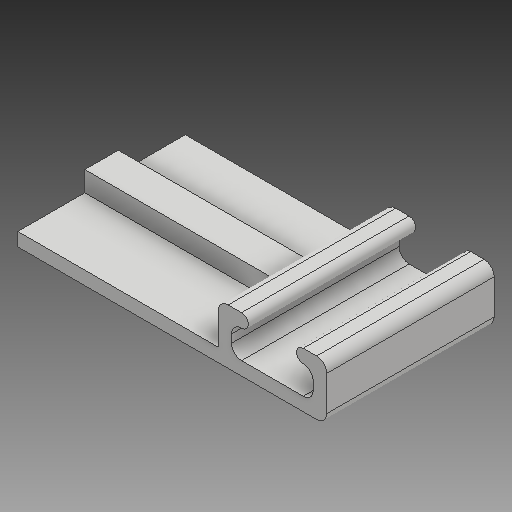
# Autodesk Inventor part: Sensor_Hook
Saved by Autodesk Inventor 2017 (Build 210142000, 142)
## iProperties
Created: 2019-10-01
Part Number: Sensor_Hook
Material: Generic
Document SubType Name: Modeling
Designer: Bear
Density: 1 g/cm^3
Appearance: Default
Author: Bear
Autodesk Inventor part; units mm, degrees
ref_plane "YZ Plane" through (0, 0, 0) normal (1, 0, 0) x (0, 1, 0)
ref_plane "XZ Plane" through (0, 0, 0) normal (0, 1, 0) x (-1, 0, 0)
ref_plane "XY Plane" through (0, 0, 0) normal (0, 0, 1) x (1, 0, 0)
sketch "Hook_Base_Skt" plane through (0, 0, 0) normal (0, 1, 0) x (-1, 0, 0)
  line L0 (4.6, -2.1) -> (-4.6, -2.1)
  line L1 (-6.1, -0.6) -> (-6.1, 0.6)
  line L2 (-4.6, 2.1) -> (4.6, 2.1) construction
  line L3 (6.1, 0.6) -> (6.1, -0.6)
  line L4 (6.1, -2.1) -> (-6.1, 2.1) construction
  line L5 (-6.1, -2.1) -> (6.1, 2.1) construction
  line L6 (8.1, -4.1) -> (-6.6, -4.1)
  line L7 (-8.1, -2.6) -> (-8.1, 2.6)
  line L8 (-6.6, 4.1) -> (-4.6, 4.1)
  line L9 (8.1, 2.6) -> (8.1, -4.1)
  line L10 (8.1, -4.1) -> (-8.1, 4.1) construction
  line L11 (-8.1, -4.1) -> (8.1, 4.1) construction
  arc A0 (6.1, 0.6) -> (4.6, 2.1) centre (4.6, 0.6) ccw
  arc A1 (4.6, -2.1) -> (6.1, -0.6) centre (4.6, -0.6) ccw
  arc A2 (-6.1, -0.6) -> (-4.6, -2.1) centre (-4.6, -0.6) ccw
  arc A3 (-4.6, 2.1) -> (-6.1, 0.6) centre (-4.6, 0.6) ccw
  arc A4 (8.1, 2.6) -> (6.6, 4.1) centre (6.6, 2.6) ccw
  arc A5 (-6.6, 4.1) -> (-8.1, 2.6) centre (-6.6, 2.6) ccw
  arc A6 (-8.1, -2.6) -> (-6.6, -4.1) centre (-6.6, -2.6) ccw
  arc A7 (4.6, 4.1) -> (4.6, 2.1) centre (4.6, 3.1) ccw
  arc A8 (-4.6, 2.1) -> (-4.6, 4.1) centre (-4.6, 3.1) ccw
  line L12 (4.6, 4.1) -> (6.6, 4.1)
  line L13 (-4.6, 4.1) -> (4.6, 4.1) construction
  point P0 (0, 0)
  dimension "d29" = 12.2
  dimension "d30" = 4.2
  dimension "d31" = 2
  dimension "d32" = 2
  dimension "d34" = 1.5
  constraints: 28 end point, 26 tangent, 18 point on circle, 14 point on line, 9 centre point, 6 equal radius, 6 parallel, 4 midpoint, 2 horizontal, 2 perpendicular
  measures "d29" distance of L4.start L5.start
  measures "d30" distance of L5.start L4.end
  measures "d31" distance between parallel lines of L9 L3
  measures "d32" distance between parallel lines of L8 L2
  measures "d34" radius of A4
extrude "Hook_Base" add sketch "Hook_Base_Skt" along normal mid plane 25
sketch "Arm_Skt" plane through (0, -12.5, 0) normal (0, -1, 0) x (1, 0, 0)
  line L0 (4.6, -2.1) -> (-4.6, -2.1) projected
  line L1 (0, -2.1) -> (-38, -2.1)
  line L2 (-38, -2.1) -> (-38, -4.1)
  line L3 (-38, -4.1) -> (0, -4.1)
  line L4 (6.6, -4.1) -> (-8.1, -4.1) projected
  line L5 (0, -4.1) -> (0, -2.1)
  point P0 (0, 0)
  dimension "d35" = 38
  constraints: 8 end point, 2 collinear, 2 perpendicular, 1 horizontal, 1 midpoint
  measures "d35" distance of L2.end L3.end
extrude "Arm" add sketch "Arm_Skt" against normal up to surface (25 mm away) from surface at 0
sketch "Arm_Rib_Skt" plane through (-38, -12.5, -2.1) normal (0, 0, 1) x (1, 0, 0)
  line L0 (38, 12.5) -> (0, 12.5) construction
  line L1 (0, 25) -> (0, 0) construction
  line L2 (29.9, 25) -> (29.9, 0) projected
  line L3 (0, 10) -> (29.9, 10)
  line L4 (29.9, 10) -> (29.9, 15)
  line L5 (29.9, 15) -> (0, 15)
  line L6 (0, 15) -> (0, 10)
  line L7 (0, 25) -> (0, 0) projected
  point P0 (0, 12.5)
  dimension "d38" = 5
  constraints: 10 end point, 3 midpoint, 2 parallel, 2 point on line, 1 horizontal, 1 perpendicular
  measures "d38" distance between parallel lines of L3 L5
extrude "Arm_Rib" add sketch "Arm_Rib_Skt" along normal blind 3
equation "\"d29\" = arm_width + 2 * clearance"
equation "\"d30\" = arm_thick + 2 * clearance"
equation "\"d31\" = hook_thick"
equation "\"d32\" = hook_thick"
equation "\"d34\" = general_fillet"
equation "\"d13\" = hook_width"
equation "\"d35\" = hole_to_border"
equation "\"d38\" = 0.2 * hook_width"
equation "\"d39\" = 1.5 * hook_thick"
equation "\"clearance\" = 0.1"
equation "\"arm_angle\" = 70deg"
equation "\"hole_diam\" = 3.1"
equation "\"hole_h_space\" = 126.2"
equation "\"hole_v_space\" = 65.65"
equation "\"arm_width\" = 12"
equation "\"arm_thick\" = 4"
equation "\"arm_rib_space\" = 1.25"
equation "\"arm_rib_thick\" = 2"
equation "\"base_width\" = 53"
equation "\"base_lenght\" = 138.2"
equation "\"general_fillet\" = 1.5"
equation "\"hole_to_border\" = 38"
equation "\"hook_width\" = 25"
equation "\"hook_thick\" = 2"
equation "\"rfid_width\" = 39.5"
equation "\"rfid_pin_border\" = 8"
equation "\"rfid_pin_width\" = 5"
equation "\"rfid_screw_h\" = 2.5"
equation "\"rfid_screw_v\" = 15.5"
equation "\"rfid_screw_diam\" = 3.1"
equation "\"rfid_clock_pad\" = 3"
equation "\"rfid_clock_h\" = 4.5"
equation "\"rfid_clock_v\" = 8.5"
equation "\"rfid_clock_thick\" = 1.5"
equation "\"finger_width\" = 21"
equation "\"finger_claw_h\" = 8"
equation "\"finger_claw_pad\" = 14"
equation "\"finger_claw_v\" = 7.3"
equation "\"finger_claw_clip\" = 2"
equation "\"finger_claw_ramp\" = 1"
body "Solid1"
